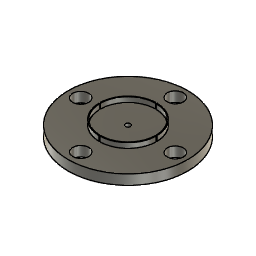
kolowybieraka v1 (Autodesk Fusion 360 design; units mm, degrees)
Autodesk Fusion 360 part; units mm, degrees
sketch "Szkic1" plane through (0, 0, 0) normal (0, 0, 1) x (1, 0, 0)
  circle A0 centre (0, 0) radius 60
  constraint coincident A0.centre origin
extrude "Wyciągnięcie proste1" add sketch "Szkic1" along normal blind 7
sketch "Szkic2" plane through (0, 0, 7) normal (0, 0, 1) x (-1, 0, 0)
  circle A0 centre (0, 0) radius 60
  line L0 (60, 0) -> (47.5, 0)
  line L1 (-47.5, 0) -> (-60, 0)
  line L2 (0.4052, -47.9052) -> (0.4052, -60.4052)
  line L3 (0.4052, 59.5948) -> (0.4052, 47.0948)
  circle A1 centre (47.5, 0) radius 7.5
  circle A2 centre (0.4052, -47.9052) radius 7.5
  circle A3 centre (-47.5, 0) radius 7.5
  circle A4 centre (0.4052, 47.0948) radius 7.5
  dimension "d3" = 12.5
  dimension "d4" = 12.5
  dimension "d5" = 12.5
  dimension "d6" = 12.5
  dimension "d7" = 15
  dimension "d8" = 15
  constraint coincident A0 L0.start
  constraint horizontal L0
  constraint horizontal L1
  constraint coincident L0.end A1.centre
  constraint coincident L2.start A2.centre
  constraint coincident L1.start A3.centre
  constraint coincident L3.end A4.centre
  measures "d3" distance of L0.start L0.end
  measures "d4" distance of L1.end L1.start
  measures "d5" distance of L2.start L2.end
  measures "d6" distance of L3.start L3.end
  measures "d7" diameter of A2
  measures "d8" diameter of A4
extrude "Wyciągnięcie proste2" cut sketch "Szkic2" against normal blind 10 contours A1 | A2 | A3 | A4
sketch "Szkic3" plane through (0, 0, 0) normal (0, 0, -1) x (1, 0, 0)
  circle A0 centre (-47.5, 0) radius 7.5
  circle A1 centre (-0.4052, 47.0948) radius 7.5
  circle A2 centre (-0.4052, -47.9052) radius 7.5
  circle A3 centre (47.5, 0) radius 7.5
  circle A4 centre (0, 0) radius 60
  circle A5 centre (0, 0) radius 2.5
  line L0 (0, 0) -> (1.5, 0)
  line L1 (1.5, 0) -> (1.5, 2.5)
  line L2 (1.5, 2.5) -> (0, 2.5)
  line L3 (0, 2.5) -> (0, 0)
  line L4 (1.5, 2.5) -> (-1.5, 2.5)
  line L5 (-1.5, 2.5) -> (-1.5, -2.5)
  line L6 (-1.5, -2.5) -> (1.5, -2.5)
  line L7 (1.5, -2.5) -> (1.5, 2.5)
  dimension "d11" = 5
  dimension "d12" = 1.5
  dimension "d13" = 2.5
  dimension "d14" = 3
  dimension "d15" = 5
  constraint coincident A4.centre A5.centre
  constraint horizontal L0
  constraint vertical L1
  constraint horizontal L2
  constraint vertical L3
  constraint horizontal L4
  constraint vertical L5
  constraint horizontal L6
  constraint vertical L7
  measures "d11" diameter of A5
  measures "d12" distance of A4.centre L0.end
  measures "d13" distance of A4.centre L2.end
  measures "d14" distance of L1.end L4.end
  measures "d15" distance of L1.end L6.end
extrude "Wyciągnięcie proste3" add sketch "Szkic3" against normal blind 10 contours A5 L0 L1 L3 L7 | A5 L0 L3 L5 L7
extrude "Wyciągnięcie proste4" cut 1 faces at (-0.3999, 0.6022, 10) along direction (0, 0, -1) blind 12
move_face "Odsuń powierzchnie1" offset 1 1 faces at (-1.403, -2.0692, 2.3333)
move_face "Odsuń powierzchnie2" offset 1 1 faces at (-1.3028, 2.1337, 4.6667)
move_face "Odsuń powierzchnie3" offset 2.5 1 faces at (-1.4925, 0.1494, 2.3333)
move_face "Odsuń powierzchnie4" offset -0.5 4 faces at (-54.9907, 0.3738, 4.6667) (-7.8679, -47.8416, 4.6667) (40.0373, 0.7468, 2.3333) (-7.8679, 47.1584, 4.6667)
sketch "Szkic4" plane through (0, 0, 7) normal (0, 0, 1) x (-1, 0, 0)
  circle A0 centre (47.5, 0) radius 8
  circle A1 centre (0.4052, 47.0948) radius 8
  circle A2 centre (0.4052, -47.9052) radius 8
  circle A3 centre (-47.5, 0) radius 8
  circle A4 centre (0, 0) radius 60
  circle A5 centre (0, 0) radius 2.5
  constraint coincident A4.centre A5.centre
extrude "Wyciągnięcie proste5" cut sketch "Szkic4" against normal blind 13 contours A5
sketch "Szkic5" plane through (0, 0, 7) normal (0, 0, 1) x (-1, 0, 0)
  circle A0 centre (0, 0) radius 2.5
  circle A1 centre (47.5, 0) radius 8
  circle A2 centre (0.4052, 47.0948) radius 8
  circle A3 centre (0.4052, -47.9052) radius 8
  circle A4 centre (-47.5, 0) radius 8
  circle A5 centre (0, 0) radius 60
  line L0 (0, 0) -> (39.5, 0)
  line L1 (39.5, 0) -> (36, 0)
  line L2 (36, 0) -> (20.5, 0)
  line L3 (36, 0) -> (28.65, 0)
  line L4 (28.65, 0) -> (27.85, 0)
  circle A6 centre (0, 0) radius 27.85
  circle A7 centre (0, 0) radius 28.65
  dimension "d26" = 15.5
  dimension "d27" = 7.35
  dimension "d28" = 0.8
  constraint coincident A0.centre A5.centre
  constraint coincident A1 L0.end
  constraint horizontal L0
  constraint coincident L0 L1.end
  constraint parallel L0 L2
  constraint coincident L2 L3.end
  constraint coincident L2 L4.end
  constraint coincident L4.end A6
  constraint coincident L3.end A7
  measures "d26" distance of L1.end L2.end
  measures "d27" distance of L1.end L3.end
  measures "d28" distance of L3.end L4.end
extrude "Wyciągnięcie proste6" add sketch "Szkic5" along normal blind 5 contours A7
sketch "Szkic6" plane through (0, 0, 12) normal (0, 0, 1) x (-1, 0, 0)
  circle A0 centre (0, 0) radius 27.85
  circle A1 centre (0, 0) radius 28.65
  line L0 (0, 0) -> (28.65, 0)
  line L1 (0, 0) -> (-28.65, 0)
  line L2 (0, 0) -> (0, -28.65)
  line L3 (0, 0) -> (0, 28.65)
  line L4 (28.65, 0) -> (27.5, 0)
  line L5 (27.5, 0) -> (27.5, -0.5)
  line L6 (27.5, -0.5) -> (28.65, -0.5)
  line L7 (28.65, -0.5) -> (28.65, 0)
  line L8 (27.5, -0.5) -> (29, -0.5)
  line L9 (29, -0.5) -> (29, 0.5)
  line L10 (29, 0.5) -> (27.5, 0.5)
  line L11 (27.5, 0.5) -> (27.5, -0.5)
  line L12 (0, 28.65) -> (-0.5, 28.65)
  line L13 (-0.5, 28.65) -> (-0.5, 27.5)
  line L14 (-0.5, 27.5) -> (0, 27.5)
  line L15 (0, 27.5) -> (0, 28.65)
  line L16 (-0.5, 27.5) -> (0.5, 27.5)
  line L17 (0.5, 27.5) -> (0.5, 29.1)
  line L18 (0.5, 29.1) -> (-0.5, 29.1)
  line L19 (-0.5, 29.1) -> (-0.5, 27.5)
  line L20 (-28.65, 0) -> (-27.5, 0)
  line L21 (-27.5, 0) -> (-27.5, -0.5)
  line L22 (-27.5, -0.5) -> (-28.65, -0.5)
  line L23 (-28.65, -0.5) -> (-28.65, 0)
  line L24 (-27.5, -0.5) -> (-29, -0.5)
  line L25 (-29, -0.5) -> (-29, 0.5)
  line L26 (-29, 0.5) -> (-27.5, 0.5)
  line L27 (-27.5, 0.5) -> (-27.5, -0.5)
  line L28 (0, -28.65) -> (0.5, -28.65)
  line L29 (0.5, -28.65) -> (0.5, -27.5)
  line L30 (0.5, -27.5) -> (0, -27.5)
  line L31 (0, -27.5) -> (0, -28.65)
  line L32 (0.5, -27.5) -> (-0.5, -27.5)
  line L33 (-0.5, -27.5) -> (-0.5, -29)
  line L34 (-0.5, -29) -> (0.5, -29)
  line L35 (0.5, -29) -> (0.5, -27.5)
  constraint coincident A0.centre A1.centre
  constraint coincident A1 L0.end
  constraint horizontal L0
  constraint coincident A1 L1.end
  constraint parallel L0 L1
  constraint coincident A1 L2.end
  constraint perpendicular L0 L2
  constraint coincident A1 L3.end
  constraint perpendicular L0 L3
  constraint horizontal L4
  constraint vertical L5
  constraint horizontal L6
  constraint vertical L7
  constraint horizontal L8
  constraint vertical L9
  constraint horizontal L10
  constraint vertical L11
  constraint horizontal L12
  constraint vertical L13
  constraint horizontal L14
  constraint vertical L15
  constraint horizontal L16
  constraint vertical L17
  constraint horizontal L18
  constraint vertical L19
  constraint horizontal L20
  constraint vertical L21
  constraint horizontal L22
  constraint vertical L23
  constraint horizontal L24
  constraint vertical L25
  constraint horizontal L26
  constraint vertical L27
  constraint horizontal L28
  constraint vertical L29
  constraint horizontal L30
  constraint vertical L31
  constraint horizontal L32
  constraint vertical L33
  constraint horizontal L34
  constraint vertical L35
extrude "Wyciągnięcie proste7" cut sketch "Szkic6" against normal blind 5 contours A0 A1 L0 L4 L6 L8 | A0 A1 L0 L4 L10 | A0 A1 L3 L15 L17 | A0 A1 L2 L29 L31 L35 | A0 A1 L3 L13 L15 L19 | A0 A1 L2 L31 L33 | A0 A1 L1 L20 L26 | A0 A1 L1 L20 L22 L24
extrude "Wyciągnięcie proste8" add 1 faces at (-16.111, 16.0947, 0) along direction (0, 0, -1) blind 3
sketch "Szkic7" plane through (0, 0, -3) normal (0, 0, -1) x (1, 0, 0)
  circle A0 centre (0, 0) radius 2.5
  circle A1 centre (-47.5, 0) radius 8
  circle A2 centre (-0.4052, 47.0948) radius 8
  circle A3 centre (-0.4052, -47.9052) radius 8
  circle A4 centre (47.5, 0) radius 8
  circle A5 centre (0, 0) radius 60
  circle A6 centre (0, 0) radius 17.5
  circle A7 centre (0, 0) radius 26
  dimension "d35" = 35
  dimension "d36" = 52
  constraint coincident A0.centre A5.centre
  measures "d35" diameter of A6
  measures "d36" diameter of A7
extrude "Wyciągnięcie proste9" cut sketch "Szkic7" against normal blind 2.5 contours A7
sketch "Szkic8" plane through (0, 0, -3) normal (0, 0, -1) x (1, 0, 0)
  circle A0 centre (0, 0) radius 60
  circle A1 centre (47.5, 0) radius 8
  circle A2 centre (-0.4052, -47.9052) radius 8
  circle A3 centre (-0.4052, 47.0948) radius 8
  circle A4 centre (-47.5, 0) radius 8
  circle A5 centre (0, 0) radius 26
